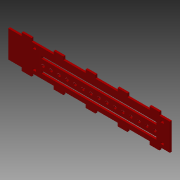
# Autodesk Inventor part: Panel3
Saved by Autodesk Inventor 2015 SP1 (Build 190203100, 203)
## iProperties
Created: 2014-08-06
Part Number: Panel3
Material: Acrylic
Document SubType Name: Modeling
Designer: Patrick Camilleri
Density: 1.188 g/cm^3
Appearance: Smooth - Red
Author: Patrick Camilleri
Autodesk Inventor part; units mm, degrees
ref_plane "YZ Plane" through (0, 0, 0) normal (1, 0, 0) x (0, 1, 0)
ref_plane "XZ Plane" through (0, 0, 0) normal (0, 1, 0) x (-1, 0, 0)
ref_plane "XY Plane" through (0, 0, 0) normal (0, 0, 1) x (1, 0, 0)
sketch "Sketch1" plane through (0, 0, 0) normal (0, 1, 0) x (-1, 0, 0)
  line L0 (21.15, 141.95) -> (-21.15, 141.95)
  line L1 (-21.15, 141.95) -> (-21.15, -110.95)
  line L2 (-21.15, -110.95) -> (21.15, -110.95)
  line L3 (21.15, -110.95) -> (21.15, 141.95)
  line L4 (21.15, 0) -> (-21.15, 0) construction
  line L5 (0, -110.95) -> (0, 141.95) construction
  point P0 (0, 0)
  point P1 (0, 0)
  dimension "d57" = 42.3
  dimension "d58" = 110.95
  dimension "d59" = 141.95
  constraints: 12 end point, 3 midpoint, 2 parallel, 2 perpendicular, 2 point on line, 1 coincident, 1 horizontal
  measures "d57" distance of L1.end L2.end
  measures "d58" distance between parallel lines of L4 L2
  measures "d59" distance between parallel lines of L4 L0
extrude "Extrusion1" add sketch "Sketch1" along normal blind 3
sketch "Sketch3" plane through (0, 0, 0) normal (0, -1, 0) x (1, 0, 0)
  line L0 (21.15, -110.95) -> (-21.15, -110.95) projected
  line L1 (21.15, 141.95) -> (21.15, -110.95) projected
  line L2 (-21.15, -110.95) -> (-21.15, 141.95) projected
  line L3 (-26.15, -79.15) -> (-21.15, -79.15)
  line L4 (-21.15, -79.15) -> (-21.15, -94.45)
  line L5 (-21.15, -94.45) -> (-26.15, -94.45)
  line L6 (-26.15, -94.45) -> (-26.15, -79.15)
  line L7 (-26.15, -79.15) -> (-21.15, -94.45) construction
  line L8 (-21.15, -79.15) -> (-26.15, -94.45) construction
  line L9 (26.15, -94.45) -> (21.15, -94.45)
  line L10 (21.15, -94.45) -> (21.15, -79.15)
  line L11 (21.15, -79.15) -> (26.15, -79.15)
  line L12 (26.15, -79.15) -> (26.15, -94.45)
  line L13 (26.15, -94.45) -> (21.15, -79.15) construction
  line L14 (21.15, -94.45) -> (26.15, -79.15) construction
  point P0 (0, 0)
  point P1 (-23.65, -86.8)
  point P2 (23.65, -86.8)
  point P3 (21.15, -86.8)
  dimension "d61" = 15.3
  dimension "d64" = 5
  dimension "d65" = 15.3
  dimension "d78" = 24.15
  dimension "d79" = 24.15
  dimension "d97" = 5
  constraints: 24 end point, 5 midpoint, 4 parallel, 2 horizontal, 2 perpendicular, 2 point on line
  measures "d61" distance of L3.end L4.end
  measures "d64" distance of L10.end L11.end
  measures "d65" distance of L9.end L10.end
  measures "d78" distance from line of L0 point (-23.65, -86.8)
  measures "d79" distance from line of L0 point (23.65, -86.8)
  measures "d97" distance between parallel lines of L6 L4
extrude "Extrusion3" add sketch "Sketch3" against normal blind 3
pattern_linear "Rectangular Pattern1" count 5 spacing 50 along (0, 0, 1) of "Extrusion3"
sketch "Sketch8" plane through (0, 3, 0) normal (0, 1, 0) x (1, 0, 0)
  line L0 (-10, -90) -> (-6, -90)
  line L1 (-6, -90) -> (-6, 90)
  line L2 (-6, 90) -> (-10, 90)
  line L3 (-10, 90) -> (-10, -90)
  line L4 (-10, -90) -> (-6, 90) construction
  line L5 (-6, -90) -> (-10, 90) construction
  line L6 (10, 90) -> (14, 90)
  line L7 (14, 90) -> (14, -90)
  line L8 (14, -90) -> (10, -90)
  line L9 (10, -90) -> (10, 90)
  line L10 (21.15, 110.95) -> (-21.15, 110.95) projected
  point P0 (-8, 0)
  dimension "d82" = 4
  dimension "d83" = 180
  dimension "d106" = 4
  dimension "d112" = 20
  constraints: 20 end point, 4 parallel, 2 horizontal, 2 midpoint, 2 perpendicular
  measures "d82" distance of L2.end L1.end
  measures "d83" distance of L1.end L0.end
  measures "d106" distance of L7.end L8.end
  measures "d112" distance between parallel lines of L3 L9
extrude "Extrusion5" cut sketch "Sketch8" against normal through all
sketch "Sketch10" plane through (0, 3, 0) normal (0, 1, 0) x (1, 0, 0)
  line L0 (10, 90) -> (14, 90) projected
  circle A0 centre (2.5, 87.5) radius 2.5
  line L1 (10, -90) -> (10, 90) projected
  point P0 (0, 0)
  dimension "d127" = 5
  dimension "d128" = 7.5
  dimension "d129" = 2.5
  constraints: 1 centre point
  measures "d127" diameter of A0
  measures "d128" distance from line of A0.centre L1
  measures "d129" distance from line of A0.centre L0
extrude "Extrusion7" cut sketch "Sketch10" against normal blind 10
pattern_linear "Rectangular Pattern6" count 15 spacing 12.5 along (0, 0, 1) of "Extrusion7"
sketch "Sketch11" plane through (0, 3, 0) normal (0, 1, 0) x (1, 0, 0)
  line L0 (21.15, 110.95) -> (-21.15, 110.95) projected
  line L1 (-21.15, 110.95) -> (-21.15, 94.45) projected
  line L2 (21.15, 94.45) -> (21.15, 110.95) projected
  line L3 (-16.15, 96.45) -> (-13.15, 96.45)
  line L4 (-13.15, 96.45) -> (-13.15, 101.45)
  line L5 (-13.15, 101.45) -> (-16.15, 101.45)
  line L6 (-16.15, 101.45) -> (-16.15, 96.45)
  line L7 (-16.15, 96.45) -> (-13.15, 101.45) construction
  line L8 (-13.15, 96.45) -> (-16.15, 101.45) construction
  line L9 (13.15, 96.45) -> (16.15, 96.45)
  line L10 (16.15, 96.45) -> (16.15, 101.45)
  line L11 (16.15, 101.45) -> (13.15, 101.45)
  line L12 (13.15, 101.45) -> (13.15, 96.45)
  line L13 (13.15, 96.45) -> (16.15, 101.45) construction
  line L14 (16.15, 96.45) -> (13.15, 101.45) construction
  point P0 (0, 0)
  point P1 (-14.65, 98.95)
  point P2 (14.65, 98.95)
  dimension "d136" = 3
  dimension "d137" = 5
  dimension "d138" = 3
  dimension "d139" = 5
  dimension "d140" = 12
  dimension "d147" = 6.5
  dimension "d148" = 6.5
  constraints: 24 end point, 4 midpoint, 4 parallel, 2 horizontal, 2 perpendicular, 1 point on line
  measures "d136" distance of L5.end L4.end
  measures "d137" distance of L4.end L3.end
  measures "d138" distance of L11.end L10.end
  measures "d139" distance of L9.end L10.end
  measures "d140" distance from line of L0 point (-14.65, 98.95)
  measures "d147" distance from line of point (-14.65, 98.95) L1
  measures "d148" distance from line of L2 point (14.65, 98.95)
extrude "Extrusion8" cut sketch "Sketch11" against normal blind 10
pattern_linear "Rectangular Pattern7" count 2 spacing 200 along (0, 0, 1) of "Extrusion8"
equation "\"d79\" = d78"
equation "\"kerf\" = 0.15"
body "Solid1"
